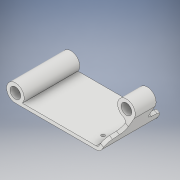
# Autodesk Inventor part: Turret Sensor Mount
Saved by Autodesk Inventor 2019.4 (Build 234330000, 330)
## iProperties
Created: 2020-01-25
Part Number: Turret Sensor Mount
Material: ABS Plastic
Document SubType Name: Modeling
Designer: admin
Density: 1.95534 g/cm^3
Appearance: Smooth - White
Mass: 200 g
Surface Area: 460.142 cm^2
Volume: 112.905 cm^3
Author: admin
Autodesk Inventor part; units mm, degrees
ref_plane "YZ Plane" through (0, 0, 0) normal (1, 0, 0) x (0, 1, 0)
ref_plane "XZ Plane" through (0, 0, 0) normal (0, 1, 0) x (-1, 0, 0)
ref_plane "XY Plane" through (0, 0, 0) normal (0, 0, 1) x (1, 0, 0)
sketch "Sketch1" plane through (0, 0, 0) normal (0, 0, 1) x (1, 0, 0)
  circle A0 centre (0, 0) radius 7.7
  circle A1 centre (0, 0) radius 12.7
  line L0 (0, 0) -> (134.976, 0) construction
  line L1 (134.976, 0) -> (134.976, 34.9) construction
  circle A2 centre (134.976, 34.9) radius 7.7
  circle A3 centre (134.976, 34.9) radius 12.7
  line L2 (0, 0) -> (134.976, 34.9) construction
  dimension "d0" = 15.4
  dimension "d3" = 5
  dimension "d13" = 15.4
  dimension "d14" = 5
  dimension "d15" = 34.9
  dimension "d16" = 139.415
  constraints: 6 end point, 4 centre point, 4 coincident, 1 horizontal, 1 vertical
  measures "d0" diameter of A0
  measures "d3" radial gap between concentric circles of A0 A1
  measures "d13" diameter of A2
  measures "d14" radial gap between concentric circles of A3 A2
  measures "d15" distance of L0.end L1.end
  measures "d16" distance of L0.start L2.end
extrude "Extrusion1" add sketch "Sketch1" along normal blind 80
sketch "Sketch3" plane through (0, 0, 80) normal (0, 0, 1) x (1, 0, 0)
  circle A0 centre (0, 0) radius 12.7 projected
  line L0 (119.2721, -7.7) -> (136.5947, 22.3036)
  circle A1 centre (134.976, 34.9) radius 12.7 projected
  line L1 (0, -12.7) -> (122.1589, -12.7)
  line L2 (122.1589, -12.7) -> (145.9746, 28.55)
  line L3 (119.2721, -7.7) -> (10.0995, -7.7)
  point P0 (0, 12.7)
  dimension "d18" = 5
  dimension "d24" = 5
  dimension "d25" = 120
  constraints: 8 end point, 5 point on circle, 2 horizontal, 2 tangent, 1 parallel
  measures "d18" distance between parallel lines of L2 L0
  measures "d24" distance between parallel lines of L1 L3
  measures "d25" angle of L3 L0
extrude "Extrusion3" add sketch "Sketch3" against normal up to surface (80 mm away) contours A0 L3 L0 A1 L2 L1
fillet "Fillet2" radius 5 3 edges at (136.5947, 22.3036, 40) (119.2721, -7.7, 40) (0, -12.7, 40)
fillet "Fillet3" radius 10 1 edges at (122.1589, -12.7, 40)
sketch "Sketch4" plane through (145.9746, 28.55, 80) normal (0.8660254, -0.5, 0) x (0, 0, -1)
  line L0 (80, -41.8579) -> (80, -17.4929) projected
  line L1 (80, -29.6754) -> (55, -24.6754)
  line L2 (55, -24.6754) -> (55, 12.7)
  line L3 (55, 12.7) -> (25, 12.7)
  line L4 (80, 12.7) -> (0, 12.7) projected
  line L5 (25, 12.7) -> (25, -24.6754)
  line L6 (25, -24.6754) -> (0, -29.6754)
  line L7 (0, -41.8579) -> (0, 0) projected
  line L8 (80, -29.6754) -> (80, 12.7)
  line L9 (80, 12.7) -> (55, 12.7)
  line L10 (25, 12.7) -> (0, 12.7)
  line L11 (0, -29.6754) -> (0, 12.7)
  point P0 (80, -97.7123)
  point P1 (40, 12.7)
  dimension "d26" = 5
  dimension "d27" = 30
  dimension "d29" = 5
  constraints: 18 end point, 3 midpoint, 2 collinear, 2 parallel, 2 perpendicular, 2 point on line, 2 vertical
  measures "d26" vertical distance of L1.start L1.end
  measures "d27" distance between parallel lines of L5 L2
  measures "d29" vertical distance of L5.end L6.end
extrude "Extrusion4" cut sketch "Sketch4" against normal through all
fillet "Fillet4" radius 10 4 edges at (128.9718, 4.1004, 0) (131.4718, 8.4305, 25) (131.4718, 8.4305, 55) (128.9718, 4.1004, 80)
sketch "Sketch5" plane through (0, -12.7, 0) normal (0, -1, 0) x (1, 0, 0)
  circle A0 centre (108.3854, 17.851) radius 2.5
  circle A1 centre (108.3854, 62.149) radius 2.5
  line L0 (108.3854, 62.149) -> (108.3854, 17.851) construction
  line L1 (108.3854, 40) -> (116.3854, 40) construction
  line L2 (116.3854, 0) -> (116.3854, 80) projected
  point P0 (0, 0)
  dimension "d33" = 5
  dimension "d34" = 5
  dimension "d35" = 44.298
  dimension "d36" = 8
  constraints: 4 end point, 2 centre point, 2 midpoint, 2 perpendicular
  measures "d33" diameter of A0
  measures "d34" diameter of A1
  measures "d35" distance of L0.start L0.end
  measures "d36" distance between parallel lines of L2 L0
extrude "Extrusion5" cut sketch "Sketch5" against normal through all
equation "\"d29\" = d26"
body "Solid1"
